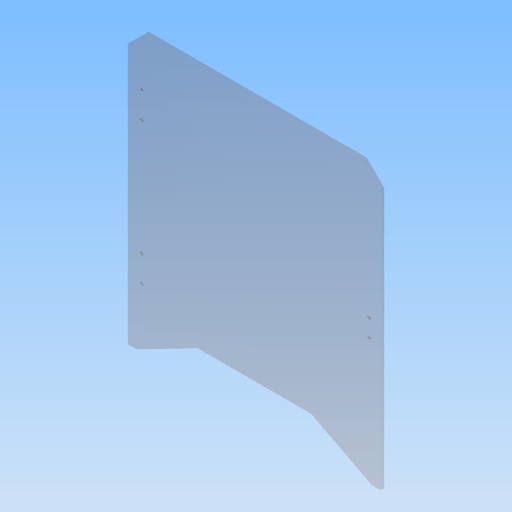
# Autodesk Inventor part: дверька
Saved by Autodesk Inventor 2017 (Build 210142000, 142)
## iProperties
Part Number: дверька
Material: Типовые
Document SubType Name: Modeling
Designer: Max
Mass: 336.61 g
Surface Area: 1733.61 cm^2
Volume: 336.61 cm^3
Density: 1 g/cm^3
Appearance: Поликарбонат — дымчатый
Author: Max
Autodesk Inventor part; units mm, degrees
ref_plane "YZ Plane" through (0, 0, 0) normal (1, 0, 0) x (0, 1, 0)
ref_plane "XZ Plane" through (0, 0, 0) normal (0, 1, 0) x (-1, 0, 0)
ref_plane "XY Plane" through (0, 0, 0) normal (0, 0, 1) x (1, 0, 0)
sketch "Эскиз1" plane through (0, 0, 0) normal (0, 0, 1) x (1, 0, 0)
  line L0 (-194.75, 26) -> (-144.75, 26) projected
  line L1 (-144.75, 26) -> (-144.75, 324) projected
  line L2 (-144.75, 324) -> (-124.75, 344) projected
  line L3 (-124.75, 344) -> (125.25, 344) projected
  line L4 (125.25, 344) -> (145.25, 324) projected
  line L5 (145.25, 324) -> (145.25, 26) projected
  line L6 (145.25, 26) -> (195.25, 26) projected
  line L7 (195.25, 26) -> (195.25, 534) projected
  line L8 (195.25, 534) -> (-194.75, 534) projected
  line L9 (-194.75, 534) -> (-194.75, 26) projected
  circle A0 centre (1.25, 464) radius 20.6 projected
  circle A1 centre (179.75, 255) radius 2 projected
  circle A2 centre (-179.25, 79.5) radius 2 projected
  circle A3 centre (179.75, 40) radius 1.5 projected
  circle A4 centre (-179.25, 337) radius 1.5 projected
  circle A5 centre (-179.25, 40) radius 1.5 projected
  circle A6 centre (-179.25, 308) radius 2 projected
  circle A7 centre (179.75, 292) radius 2 projected
  circle A8 centre (-158.5, 122) radius 1.5 projected
  circle A9 centre (-158.5, 254) radius 1.5 projected
  circle A10 centre (-158.5, 284) radius 1.5 projected
  circle A11 centre (-158.5, 92) radius 1.5 projected
  circle A12 centre (150.5171, 178.4783) radius 1.5 projected
  line L10 (-144.25, 26) -> (144.75, 26)
  line L11 (-124.5429, 343.5) -> (-144.25, 323.7929)
  line L12 (-144.25, 323.7929) -> (-144.25, 26)
  line L13 (-144.25, 25.5) -> (-195.25, 25.5)
  line L14 (-195.25, 25.5) -> (-195.25, 534.5)
  line L15 (-195.25, 534.5) -> (195.75, 534.5)
  line L16 (195.75, 534.5) -> (195.75, 25.5)
  line L17 (195.75, 25.5) -> (144.75, 25.5)
  line L18 (144.75, 26) -> (144.75, 323.7929)
  line L19 (144.75, 323.7929) -> (125.0429, 343.5)
  line L20 (125.0429, 343.5) -> (-124.5429, 343.5)
  circle A13 centre (-130.5, 284) radius 1.5 projected
  circle A14 centre (-130.5, 254) radius 1.5 projected
  circle A15 centre (-130.5, 122) radius 1.5 projected
  circle A16 centre (-130.5, 92) radius 1.5 projected
  dimension "d21" = 0.5
  dimension "d22" = 0.5
  dimension "d23" = 0.5
  dimension "d24" = 0.5
  constraints: 22 end point, 2 collinear, 5 other
  measures "d21" distance between parallel lines of L2 L11
  measures "d22" distance between parallel lines of L5 L18
  measures "d23" distance between parallel lines of L1 L12
  measures "d24" distance between parallel lines of L20 L3
extrude "Выдавливание1" add sketch "Эскиз1" against normal blind 4 contours L12 L11 L20 L19 L18 L10
sketch "Эскиз2" plane through (0, 0, 0) normal (0, 0, 1) x (1, 0, 0)
  circle A0 centre (-130.5, 92) radius 1.5 projected
  circle A1 centre (-130.5, 122) radius 1.5 projected
  circle A2 centre (-130.5, 254) radius 1.5 projected
  circle A3 centre (-130.5, 284) radius 1.5 projected
  line L0 (-114.5429, 343.5) -> (-144.25, 313.7929) projected
  line L1 (-144.25, 313.7929) -> (-144.25, 43.1688) projected
  line L2 (-144.25, 43.1688) -> (-103.3546, -10.5) projected
  line L3 (-103.3546, -10.5) -> (103.8544, -10.5) projected
  line L4 (103.8544, -10.5) -> (144.75, 43.1637) projected
  line L5 (144.75, 43.1637) -> (144.75, 313.7929) projected
  line L6 (144.75, 313.7929) -> (115.0429, 343.5) projected
  line L7 (115.0429, 343.5) -> (-114.5429, 343.5) projected
  line L8 (144.75, 43.1637) -> (144.75, 313.7929) projected
  line L9 (144.75, 178.4783) -> (129.75, 178.4783)
  line L10 (129.75, 178.4783) -> (129.75, 188.4783)
  circle A4 centre (129.75, 188.4783) radius 1.5
  circle A5 centre (129.75, 168.4783) radius 1.5
  point P0 (0, 0)
  dimension "d7" = 3
  dimension "d8" = 3
  dimension "d9" = 10
  dimension "d10" = 20
  dimension "d11" = 15
  constraints: 4 end point, 2 centre point, 2 perpendicular, 1 coincident, 1 midpoint
  measures "d7" diameter of A4
  measures "d8" diameter of A5
  measures "d9" distance from line of L9 L10.end
  measures "d10" distance of A5.centre L10.end
  measures "d11" distance from line of L5 A4.centre
extrude "Выдавливание2" cut sketch "Эскиз2" against normal blind 10 contours A4 | A5
sketch "Эскиз4" plane through (0, 0, 0) normal (0, 0, 1) x (1, 0, 0)
  line L0 (-106.1226, 31) -> (-137.405, 31) projected
  line L1 (137.905, 31) -> (106.6226, 31) projected
  line L2 (-103.3546, -10.5) -> (-144.25, 43.1688) projected
  line L3 (-134.9774, 31) -> (135.4804, 31)
  line L4 (144.75, 43.1637) -> (103.8544, -10.5) projected
  line L5 (-103.3546, -10.5) -> (103.8544, -10.5) projected
  line L6 (-134.9774, 31) -> (-103.3546, -10.5)
  line L7 (-103.3546, -10.5) -> (103.8544, -10.5)
  line L8 (103.8544, -10.5) -> (135.4804, 31)
  line L9 (-131.1675, 26) -> (131.67, 26)
  point P0 (0, 0)
  dimension "d16" = 0
  dimension "d19" = 12.1688
  dimension "d20" = 5
  constraints: 10 end point, 4 point on line, 3 collinear, 1 horizontal
  measures "d16" distance between parallel lines of L0 L3
  measures "d19" distance from line of L0 L2.end
  measures "d20" distance between parallel lines of L9 L3
extrude "Выдавливание4" cut sketch "Эскиз4" against normal blind 5 contours L9 L4 L5 L2
sketch "Эскиз7" plane through (0, 0, 0) normal (0, 0, 1) x (1, 0, 0)
  line L0 (-131.9699, 31.6699) -> (-66.8244, 65.3301) construction
  line L1 (-64.0309, 66) -> (0.25, 66) construction
  line L2 (0.25, 65.3301) -> (57.2313, 65.3301) construction
  line L3 (59.4686, 65.3301) -> (67.3244, 65.3301) construction
  line L4 (67.3244, 65.3301) -> (132.4699, 31.6699) construction
  line L5 (144.9404, 31) -> (68.8214, 70.3301) construction
  line L6 (-144.4404, 31) -> (-68.3214, 70.3301) construction
  line L7 (0.25, 71) -> (-65.5279, 71) construction
  line L8 (66.0279, 71) -> (0.25, 71) construction
  line L9 (-144.25, 26) -> (144.75, 26) projected
  line L10 (-134.2295, 26) -> (-64.5556, 62)
  line L11 (-64.5556, 62) -> (65.0556, 62)
  line L12 (65.0556, 62) -> (134.7295, 26)
  line L13 (134.7295, 26) -> (-134.2295, 26)
  line L14 (-144.25, 323.7929) -> (-144.25, 26) projected
  line L15 (144.75, 323.7929) -> (144.75, 26) projected
  point P0 (0, 0)
  dimension "d32" = 4
  dimension "d33" = 4
  dimension "d34" = 4
  constraints: 8 end point, 5 parallel, 2 point on line
  measures "d32" distance between parallel lines of L10 L0
  measures "d33" distance between parallel lines of L1 L11
  measures "d34" distance between parallel lines of L4 L12
extrude "Выдавливание6" cut sketch "Эскиз7" against normal blind 5
